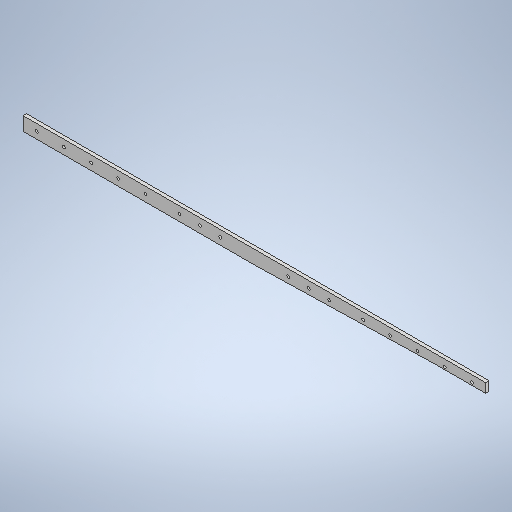
# Autodesk Inventor part: Verstärkungsstrebe
Saved by Autodesk Inventor 2025 (Build 290162000, 162)
## iProperties
Created: 2025-12-04
Part Number: Verstärkungsstrebe
Material: Generic
Document SubType Name: Modeling
Designer: ruven
Density: 1 g/cm^3
Appearance: Default
Author: ruven
Autodesk Inventor part; units mm, degrees
ref_plane "YZ Plane" through (0, 0, 0) normal (1, 0, 0) x (0, 1, 0)
ref_plane "XZ Plane" through (0, 0, 0) normal (0, 1, 0) x (-1, 0, 0)
ref_plane "XY Plane" through (0, 0, 0) normal (0, 0, 1) x (1, 0, 0)
sketch "Sketch1" plane through (0, 0, 0) normal (0, 1, 0) x (-1, 0, 0)
  line L0 (343.2337, 10.8883) -> (-336.7663, 10.8883)
  circle A0 centre (-316.7663, 0.8883) radius 2
  circle A1 centre (-276.7663, 0.8883) radius 2
  circle A2 centre (-236.7663, 0.8883) radius 2
  circle A3 centre (-196.7663, 0.8883) radius 2
  circle A4 centre (-156.7663, 0.8883) radius 2
  circle A5 centre (-106.7663, 0.8883) radius 2
  circle A6 centre (-76.7663, 0.8883) radius 2
  circle A7 centre (-46.7663, 0.8883) radius 2
  circle A8 centre (53.2337, 0.8883) radius 2
  circle A9 centre (83.2337, 0.8883) radius 2
  circle A10 centre (113.2337, 0.8883) radius 2
  circle A11 centre (163.2337, 0.8883) radius 2
  circle A12 centre (203.2337, 0.8883) radius 2
  circle A13 centre (243.2337, 0.8883) radius 2
  circle A14 centre (283.2337, 0.8883) radius 2
  circle A15 centre (323.2337, 0.8883) radius 2
  line L1 (-336.7663, 10.8883) -> (-336.7663, -9.1117)
  line L2 (-336.7663, -9.1117) -> (343.2337, -9.1117)
  line L3 (343.2337, -9.1117) -> (343.2337, 10.8883)
  line L4 (-336.7663, 10.8883) -> (343.2337, 10.8883)
  line L5 (-336.7663, 0.8883) -> (343.2337, 0.8883) construction
  point P0 (0, 0)
  point P1 (-434.8662, -18.5117)
  point P2 (3.2337, 10.8883)
  dimension "d0" = 680
  dimension "d1" = 340
  dimension "d2" = 20
  dimension "d3" = 680
  dimension "d6" = 10
  dimension "d7" = 10
  dimension "d8" = 10
  dimension "d9" = 0
  dimension "d10" = 10
  dimension "d11" = 10
  dimension "d12" = 10
  dimension "d13" = 10
  dimension "d14" = 10
  dimension "d15" = 10
  dimension "d16" = 10
  dimension "d17" = 10
  dimension "d18" = 10
  dimension "d19" = 10
  dimension "d20" = 10
  dimension "d21" = 10
  constraints: 16 centre point, 12 end point, 3 midpoint, 3 perpendicular, 2 equal length, 1 other
  measures "d0" distance from line of L5.end L1
  measures "d1" distance from line of point (3.234, 10.888) L3
  measures "d2" distance of L0.end L1.end
  measures "d3" distance of L1.end L2.end
  measures "d6" distance from line of L2 A0.centre
  measures "d7" distance from line of L0 A1.centre
  measures "d8" distance from line of L0 A2.centre
  measures "d9" distance from line of A15.centre L5
  measures "d10" distance from line of L0 A14.centre
  measures "d11" distance from line of L0 A13.centre
  measures "d12" distance from line of L0 A12.centre
  measures "d13" distance from line of L4 A11.centre
  measures "d14" distance from line of L4 A10.centre
  measures "d15" distance from line of L0 A9.centre
  measures "d16" distance from line of L0 A8.centre
  measures "d17" distance from line of L4 A7.centre
  measures "d18" distance from line of L4 A6.centre
  measures "d19" distance from line of L0 A5.centre
  measures "d20" distance from line of L0 A4.centre
  measures "d21" distance from line of L4 A3.centre
extrude "Extrusion1" add sketch "Sketch1" along normal blind 5
sketch "Sketch2" plane through (0, 0, 0) normal (0, -1, 0) x (1, 0, 0)
  line L0 (-343.2337, -9.1117) -> (-343.2337, 10.8883) projected
  line L1 (336.7663, -9.1117) -> (-343.2337, -9.1117) projected
  line L2 (336.7663, 10.8883) -> (336.7663, -9.1117) projected
  line L3 (261.2812, -2.6683) -> (0, -9.1117)
  line L4 (336.7663, -9.1117) -> (336.7663, -2.6683)
  line L5 (336.7663, -2.6683) -> (261.2812, -2.6683)
  point P0 (0, 0)
  point P1 (336.7663, -0.8068)
  constraints: 6 end point, 2 point on line, 1 collinear, 1 perpendicular
extrude "Extrusion2" cut sketch "Sketch2" against normal through all
body "Solid1"
